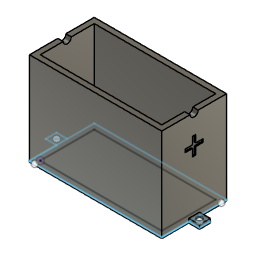
Hloder v1 (Autodesk Fusion 360 design; units mm, degrees)
Autodesk Fusion 360 part; units mm, degrees
sketch "Sketch1" plane through (0, 0, 0) normal (0, 0, 1) x (1, 0, 0)
  line L0 (0, 0) -> (0, 20)
  line L1 (0, 0) -> (45, 0)
  line L2 (45, 0) -> (45, 20)
  line L3 (45, 20) -> (0, 20)
  line L4 (47, 20) -> (47, 22)
  line L5 (0, -2) -> (-2, -2)
  line L6 (-2, -2) -> (47, -2)
  line L7 (47, -2) -> (47, 22)
  line L8 (47, 22) -> (-2, 22)
  line L9 (-2, 22) -> (-2, -2)
  line L10 (47, -2) -> (47, 8)
  line L11 (47, 8) -> (51, 8)
  line L12 (51, 8) -> (51, 12)
  line L13 (51, 12) -> (47, 12)
  circle A0 centre (49, 10) radius 1
  line L14 (-2, -2) -> (-2, 8)
  line L15 (-2, 8) -> (-6, 8)
  line L16 (-6, 8) -> (-6, 12)
  line L17 (-6, 12) -> (-2, 12)
  circle A1 centre (-4, 10) radius 1
  dimension "d1" = 20
  dimension "d2" = 45
  dimension "d3" = 2
  dimension "d20" = 10
  dimension "d21" = 4
  dimension "d22" = 4
  dimension "d23" = 2
  dimension "d24" = 10
  dimension "d25" = 4
  dimension "d26" = 4
  dimension "d27" = 2
  constraint coincident L0.start L1.start
  constraint vertical L0
  constraint perpendicular L0 L1
  constraint perpendicular L1 L2
  constraint perpendicular L0 L3
  constraint perpendicular L3 L4
  constraint perpendicular L0 L5
  constraint horizontal L6
  constraint vertical L7
  constraint horizontal L8
  constraint vertical L9
  constraint perpendicular L8 L10
  constraint perpendicular L10 L11
  constraint perpendicular L11 L12
  constraint coincident L7 L13.end
  constraint perpendicular L7 L13
  constraint perpendicular L5 L14
  constraint perpendicular L14 L15
  constraint perpendicular L15 L16
  constraint coincident L9 L17.end
  constraint perpendicular L9 L17
  measures "d1" distance of L0.start L0.end
  measures "d2" distance of L0.start L1.end
  measures "d3" distance of L2.end L4.start
  measures "d20" distance of L6.end L10.end
  measures "d21" distance of L10.end L11.end
  measures "d22" distance of L11.end L12.end
  measures "d23" diameter of A0
  measures "d24" distance of L5.end L14.end
  measures "d25" distance of L14.end L15.end
  measures "d26" distance of L15.end L16.end
  measures "d27" diameter of A1
extrude "Extrude1" add sketch "Sketch1" against normal blind 0.5 contours L0 L1 L2 L3 | L4 L5 L6 L7 L8 L9 L10 L14
extrude "Extrude2" add sketch "Sketch1" along normal blind 34 contours L4 L5 L6 L7 L8 L9 L10 L14
sketch "Sketch2" plane through (-2, 0, 0) normal (-1, 0, 0) x (0, -1, 0)
  line L0 (-22, 34) -> (-22, -0.5)
  line L1 (-22, -0.5) -> (2, -0.5)
  line L2 (2, -0.5) -> (2, 34)
  line L3 (2, 34) -> (-22, 34)
  circle A0 centre (-10, 34) radius 1.5
  line L4 (-15, 20) -> (-5, 20) construction
  line L5 (-5, 20) -> (-5, 25) construction
  line L6 (-5, 25) -> (-15, 25) construction
  line L7 (-15, 25) -> (-15, 20) construction
  dimension "d11" = 3
  dimension "d12" = 10
  text T0 "\n-" font "Arial" height 10 align centre bottom in box 10 x 5 at (-15, 20) x (1, 0) y (0, 1) spacing 1
  constraint midpoint L3 A0.centre
  measures "d11" diameter of A0
sketch "Sketch3" plane through (47, 0, 0) normal (1, 0, 0) x (0, 1, 0)
  line L0 (-2, 34) -> (-2, -0.5)
  line L1 (-2, -0.5) -> (22, -0.5)
  line L2 (22, -0.5) -> (22, 34)
  line L3 (22, 34) -> (-2, 34)
  line L4 (5, 20) -> (15, 20) construction
  line L5 (15, 20) -> (15, 25) construction
  line L6 (15, 25) -> (5, 25) construction
  line L7 (5, 25) -> (5, 20) construction
  dimension "d13" = 10
  text T0 "+" font "Arial" height 10 align centre middle in box 10 x 5 at (5, 20) x (1, 0) y (0, 1) spacing 1
extrude "Extrude3" cut sketch "Sketch3" against normal blind 0.5 text T0
extrude "Extrude4" cut sketch "Sketch2" against normal blind 0.5 text T0
extrude "Extrude5" cut sketch "Sketch2" against normal blind 49 contours L3 A0 picked at (-10.3491, 33.1105)
extrude "Extrude6" add sketch "Sketch1" against normal blind 0.5 contours L7 L11 L12 L13 | L9 L15 L16 L17
extrude "Extrude7" add sketch "Sketch1" along normal blind 1 contours L7 L11 L12 L13 | L9 L15 L16 L17
